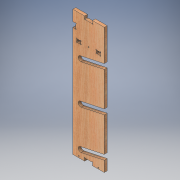
# Autodesk Inventor part: rack sides
Saved by Autodesk Inventor 2016 (Build 200138000, 138)
## iProperties
Created: 2017-03-12
Part Number: rack sides
Material: Wood (Birch)
Document SubType Name: Modeling
Designer: jwillauer
Density: 0.55 g/cm^3
Appearance: Birch - Natural Polished
Author: jwillauer
Autodesk Inventor part; units mm, degrees
ref_plane "YZ Plane" through (0, 0, 0) normal (1, 0, 0) x (0, 1, 0)
ref_plane "XZ Plane" through (0, 0, 0) normal (0, 1, 0) x (-1, 0, 0)
ref_plane "XY Plane" through (0, 0, 0) normal (0, 0, 1) x (1, 0, 0)
sketch "Sketch1" plane through (0, 0, 0) normal (0, 0, 1) x (1, 0, 0)
  line L0 (-71.8432, 70.6031) -> (131.3568, 70.6031)
  line L1 (131.3568, -742.1969) -> (-71.8432, -742.1969)
  line L2 (-71.8432, -742.1969) -> (-71.8432, 70.6031)
  line L3 (131.3568, -132.5969) -> (-10.9328, -162.8415)
  line L4 (131.3568, -165.0562) -> (-19.8283, -197.1916)
  arc A0 (-24.3438, -165.6921) -> (-17.7426, -196.7483) centre (-21.0432, -181.2202) ccw
  line L5 (131.3568, 70.6031) -> (131.3568, -132.5969)
  line L6 (131.3568, -165.0562) -> (131.3568, -742.1969) construction
  line L7 (131.3568, -386.5969) -> (-10.9328, -416.8415)
  line L8 (131.3568, -419.0562) -> (-19.8283, -451.1916)
  arc A1 (-24.3438, -419.6921) -> (-17.7426, -450.7483) centre (-21.0432, -435.2202) ccw
  line L9 (131.3568, -640.5969) -> (-10.9328, -670.8415)
  line L10 (131.3568, -673.0562) -> (-19.8283, -705.1916)
  arc A2 (-24.3438, -673.6921) -> (-17.7426, -704.7483) centre (-21.0432, -689.2202) ccw
  line L11 (131.3568, -165.0562) -> (131.3568, -386.5969)
  line L12 (131.3568, -419.0562) -> (131.3568, -640.5969)
  line L13 (131.3568, -673.0562) -> (131.3568, -742.1969)
  line L14 (-24.3438, -165.6921) -> (-10.9328, -162.8415)
  line L15 (-24.3438, -419.6921) -> (-10.9328, -416.8415)
  line L16 (-24.3438, -673.6921) -> (-9.6152, -670.5614)
  point P0 (0, 0)
  dimension "d0" = 203.2
  dimension "d1" = 812.8
  dimension "d3" = 31.75
  dimension "d4" = 203.2
  dimension "d7" = 254
  dimension "d48" = 152.4
  constraints: 34 end point, 7 point on circle, 7 point on line, 4 parallel, 3 centre point, 3 collinear, 2 perpendicular, 2 tangent, 1 horizontal, 1 vertical, 20 other
  measures "d0" distance of L0.start L0.end
  measures "d1" distance of L1.end L0.start
  measures "d3" distance between parallel lines of L3 L4
  measures "d4" distance of L0.end L3.start
  measures "d7" distance of L3.end L7.end
  measures "d48" horizontal distance of L4.start A0.centre
extrude "Extrusion1" add sketch "Sketch1" along normal blind 18.796
sketch "Sketch3" plane through (0, 0, 18.796) normal (0, 0, 1) x (1, 0, 0)
  line L0 (-71.8432, 70.6031) -> (131.3568, 70.6031) projected
  line L1 (4.3568, 70.6031) -> (55.5231, 70.6031)
  line L2 (55.5231, 70.6031) -> (55.5231, 51.8071)
  line L3 (55.5231, 51.8071) -> (4.3568, 51.8071)
  line L4 (4.3568, 51.8071) -> (4.3568, 70.6031)
  line L5 (-71.8432, 70.6031) -> (-71.8432, -742.1969) projected
  point P0 (0, 0)
  dimension "d31" = 18.796
  dimension "d32" = 0
  dimension "d34" = 76.2
  constraints: 8 end point, 2 parallel, 1 horizontal, 1 perpendicular
  measures "d31" distance between parallel lines of L1 L3
  measures "d32" distance between parallel lines of L0 L1
  measures "d34" distance between parallel lines of L5 L4
extrude "Extrusion2" cut sketch "Sketch3" against normal blind 18.796
sketch "Sketch5" plane through (0, 0, 18.796) normal (0, 0, 1) x (1, 0, 0)
  line L0 (80.5568, -81.7969) -> (105.9568, -81.7969)
  line L1 (105.9568, -81.7969) -> (105.9568, -100.5929)
  line L2 (105.9568, -100.5929) -> (80.5568, -100.5929)
  line L3 (80.5568, -100.5929) -> (80.5568, -81.7969)
  line L4 (-71.8432, 70.6031) -> (-71.8432, -742.1969) projected
  line L5 (131.3568, -132.5969) -> (131.3568, 70.6031) projected
  line L6 (131.3568, 70.6031) -> (55.5231, 70.6031) projected
  line L7 (-21.0432, -81.7969) -> (-46.4432, -81.7969)
  line L8 (-46.4432, -81.7969) -> (-46.4432, -100.5929)
  line L9 (-46.4432, -100.5929) -> (-21.0432, -100.5929)
  line L10 (-21.0432, -100.5929) -> (-21.0432, -81.7969)
  line L11 (4.3568, -742.1969) -> (55.1568, -742.1969)
  line L12 (55.1568, -742.1969) -> (55.1568, -723.4009)
  line L13 (55.1568, -723.4009) -> (4.3568, -723.4009)
  line L14 (4.3568, -723.4009) -> (4.3568, -742.1969)
  line L15 (-71.8432, -742.1969) -> (131.3568, -742.1969) projected
  point P0 (0, 0)
  dimension "d51" = 25.4
  dimension "d52" = 18.796
  dimension "d53" = 25.4
  dimension "d54" = 152.4
  dimension "d55" = 25.4
  dimension "d56" = 18.796
  dimension "d57" = 25.4
  dimension "d58" = 50.8
  dimension "d59" = 18.796
  dimension "d60" = 0
  dimension "d61" = 76.2
  constraints: 24 end point, 6 parallel, 3 horizontal, 3 perpendicular
  measures "d51" distance of L0.start L0.end
  measures "d52" distance between parallel lines of L0 L2
  measures "d53" distance between parallel lines of L5 L1
  measures "d54" distance between parallel lines of L0 L6
  measures "d55" distance of L7.start L7.end
  measures "d56" distance of L9.end L7.start
  measures "d57" distance between parallel lines of L4 L8
  measures "d58" distance of L12.end L13.end
  measures "d59" distance of L11.end L12.end
  measures "d60" distance between parallel lines of L15 L11
  measures "d61" distance between parallel lines of L4 L14
extrude "Extrusion4" cut sketch "Sketch5" against normal blind 25.4
sketch "Sketch6" plane through (0, 0, 18.796) normal (0, 0, 1) x (1, 0, 0)
  line L0 (-71.8432, 70.6031) -> (4.3568, 70.6031) projected
  line L1 (-71.8432, 1.0071) -> (-53.0472, 1.0071)
  line L2 (-71.8432, -30.9969) -> (-53.0472, -30.9969)
  line L3 (-71.8432, 1.0071) -> (-71.8432, -30.9969)
  line L4 (-71.8432, -742.1969) -> (-71.8432, 70.6031) projected
  line L5 (-53.0472, 1.0071) -> (-53.0472, -30.9969)
  point P0 (0, 0)
  dimension "d66" = 32.004
  dimension "d68" = 18.796
  constraints: 8 end point, 1 parallel, 1 perpendicular, 1 point on line
  measures "d66" distance between parallel lines of L1 L2
  measures "d68" distance between parallel lines of L5 L3
extrude "Extrusion5" cut sketch "Sketch6" against normal blind 25.4
sketch "Sketch8" plane through (0, 0, 18.796) normal (0, 0, 1) x (1, 0, 0)
  line L0 (4.3568, -742.1969) -> (4.3568, -723.4009) projected
  line L1 (4.3568, -723.4009) -> (55.1568, -723.4009) projected
  point P0 (0, 0)
  point P1 (4.3568, 51.8071)
  point P2 (55.5513, 51.8071)
hole "Hole2" at (4.3568, 51.8071, 18.796) at (55.5513, 51.8071, 18.796) at (4.3568, -723.4009, 18.796) at (55.1568, -723.4009, 18.796) direction (0, 0, -1) diameter 6.35 end through all
sketch "Sketch9" plane through (0, 0, 18.796) normal (0, 0, 1) x (1, 0, 0)
  line L0 (-21.0432, -81.7969) -> (-46.4432, -81.7969) projected
  line L1 (-21.0432, -100.5929) -> (-21.0432, -81.7969) projected
  line L2 (-46.4432, -100.5929) -> (-21.0432, -100.5929) projected
  line L3 (105.9568, -81.7969) -> (80.5568, -81.7969) projected
  line L4 (80.5568, -100.5929) -> (105.9568, -100.5929) projected
  line L5 (105.9568, -100.5929) -> (105.9568, -81.7969) projected
  point P0 (0, 0)
  point P1 (-46.6954, -81.6809)
  constraints: 2 coincident
hole "Hole3" at (-46.6954, -81.6809, 18.796) at (-21.0432, -81.7969, 18.796) at (-21.0432, -100.5929, 18.796) at (-46.4432, -100.5929, 18.796) at (80.5568, -81.7969, 18.796) at (80.5568, -100.5929, 18.796) at (105.9568, -100.5929, 18.796) at (105.9568, -81.7969, 18.796) direction (0, 0, -1) diameter 6.35 end through all
sketch "Sketch10" plane through (0, 0, 18.796) normal (0, 0, 1) x (1, 0, 0)
  line L0 (-53.0472, 1.0071) -> (-71.8432, 1.0071) projected
  point P0 (0, 0)
  point P1 (-53.0472, -31.6336)
hole "Hole4" at (-53.0472, 1.0071, 18.796) at (-53.0472, -31.6336, 18.796) direction (0, 0, -1) diameter 6.35 end through all
sketch "Sketch11" plane through (0, 0, 18.796) normal (0, 0, 1) x (1, 0, 0)
  line L0 (-71.8432, -30.9969) -> (-71.8432, -742.1969) projected
  line L1 (55.1568, -726.5759) -> (55.1568, -742.1969) projected
  line L2 (131.3568, -742.1969) -> (131.3568, -673.0562) projected
  point P0 (0, 0)
  point P1 (29.7568, -91.1319)
  point P2 (-33.7432, -732.2316)
  point P3 (55.1568, -734.3864)
  point P4 (93.2568, -734.3864)
  dimension "d92" = 101.6
  dimension "d93" = 38.1
  dimension "d94" = 38.1
  constraints: 1 midpoint
  measures "d92" distance from line of L0 point (29.757, -91.132)
  measures "d93" distance from line of L2 point (93.257, -734.386)
  measures "d94" distance from line of L0 point (-33.743, -732.232)
hole "Hole5" at (29.7568, -91.1319, 18.796) at (-33.7432, -732.2316, 18.796) at (55.1568, -734.3864, 18.796) at (93.2568, -734.3864, 18.796) direction (0, 0, -1) diameter 6.35 end through all
body "Solid1"
